# Autodesk Inventor part: JP1_1X06_NO_SILK
Saved by Autodesk Inventor 2016 SP1 (Build 200210100, 210)
## iProperties
Created: 2015-11-19
Part Number: JP1_1X06_NO_SILK
Material: Generic
Document SubType Name: Modeling
Designer: PhillipD
Density: 1 g/cm^3
Appearance: 1X06_NO_SILK, JP1_1X06_NO_SILK
Author: PhillipD
Autodesk Inventor part; units mm, degrees
ref_plane "YZ Plane" through (0, 0, 0) normal (1, 0, 0) x (0, 1, 0)
ref_plane "XZ Plane" through (0, 0, 0) normal (0, 1, 0) x (-1, 0, 0)
ref_plane "XY Plane" through (0, 0, 0) normal (0, 0, 1) x (1, 0, 0)
sketch "1X06_NO_SILK, JP1_1X06_NO_SILK_24" plane through (0, 0, 0) normal (0, 0, 1) x (1, 0, 0)
  line L0 (-0.254, 0.254) -> (12.954, 0.254)
  line L1 (12.954, 0.254) -> (12.954, -0.254)
  line L2 (12.954, -0.254) -> (-0.254, -0.254)
  line L3 (-0.254, -0.254) -> (-0.254, 0.254)
  constraints: 8 end point
extrude "Extrusion1" add sketch "1X06_NO_SILK, JP1_1X06_NO_SILK_24" along normal blind 1
body "Solid1"
